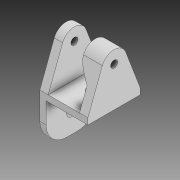
# Autodesk Inventor part: ZIdler
Saved by Autodesk Inventor 2020 (Build 240168000, 168)
## iProperties
Created: 2020-10-21
Part Number: ZIdler
Material: Generic
Document SubType Name: Modeling
Designer: DDeGo
Density: 1 g/cm^3
Appearance: Default
Author: DDeGo
Autodesk Inventor part; units mm, degrees
ref_plane "YZ Plane" through (0, 0, 0) normal (1, 0, 0) x (0, 1, 0)
ref_plane "XZ Plane" through (0, 0, 0) normal (0, 1, 0) x (-1, 0, 0)
ref_plane "XY Plane" through (0, 0, 0) normal (0, 0, 1) x (1, 0, 0)
sketch "Sketch1" plane through (0, 0, 0) normal (0, 0, 1) x (1, 0, 0)
  line L0 (0, 0) -> (23, 0)
  line L1 (23, 0) -> (23, -3)
  line L2 (23, -3) -> (3, -3)
  line L3 (3, -3) -> (3, -23)
  line L4 (3, -23) -> (0, -23)
  line L5 (0, -23) -> (0, 0)
  dimension "d0" = 3
  dimension "d1" = 20
  constraints: 12 end point, 7 perpendicular, 1 horizontal
  measures "d0" distance of L0.end L1.end
  measures "d1" distance of L1.end L2.end
extrude "Extrusion1" add sketch "Sketch1" along normal mid plane 25
sketch "Sketch2" plane through (0, 0, 12.5) normal (0, 1, 0) x (1, 0, 0)
  line L0 (23, 25) -> (23, 0) projected
  line L1 (23, 12.5) -> (13, 12.5) construction
  circle A0 centre (13, 12.5) radius 2.75
  line L2 (3, 25) -> (3, 0) projected
  dimension "d14" = 10
  dimension "d15" = 5.5
  constraints: 2 end point, 1 centre point, 1 coincident, 1 horizontal, 1 midpoint
  measures "d14" distance from line of L2 L1.end
  measures "d15" diameter of A0
extrude "Extrusion2" cut sketch "Sketch2" against normal through all
sketch "Sketch3" plane through (0, -23, 12.5) normal (-1, 0, 0) x (0, 0, 1)
  line L0 (-25, 0) -> (0, 0) projected
  line L1 (-12.5, 0) -> (-12.5, 10) construction
  circle A0 centre (-12.5, 10) radius 2.75
  line L2 (-25, 20) -> (0, 20) projected
  point P0 (-12.5, 23)
  dimension "d10" = 10
  dimension "d11" = 5.5
  constraints: 2 end point, 1 centre point, 1 coincident, 1 midpoint, 1 vertical
  measures "d10" distance from line of L1.end L2
  measures "d11" diameter of A0
extrude "Extrusion3" cut sketch "Sketch3" against normal through all
sketch "Sketch5" plane through (0, -23, 12.5) normal (-1, 0, 0) x (0, 0, 1)
  line L0 (-12.5, 23) -> (-12.5, 39) construction
  arc A0 (-6.8914, 41.1317) -> (-18.1086, 41.1317) centre (-12.5, 39) ccw
  circle A1 centre (-12.5, 39) radius 1.65
  line L1 (-25, 23) -> (0, 23) projected
  line L2 (-25, 23) -> (-18.1086, 41.1317)
  line L3 (-6.8914, 41.1317) -> (0, 23)
  line L4 (0, 23) -> (-25, 23)
  dimension "d23" = 3.3
  dimension "d24" = 12
  dimension "d25" = 16
  constraints: 8 end point, 2 centre point, 2 coincident, 2 point on circle, 2 tangent, 1 collinear, 1 vertical
  measures "d23" diameter of A1
  measures "d24" diameter of A0
  measures "d25" distance of L0.start L0.end
extrude "Extrusion5" add sketch "Sketch5" against normal blind 4
sketch "Sketch6" plane through (23, -3, 12.5) normal (1, 0, 0) x (0, 0, -1)
  line L0 (6.8914, 21.1317) -> (0, 3) projected
  line L1 (25, 3) -> (0, 3) projected
  line L2 (25, 3) -> (18.1086, 21.1317) projected
  arc A0 (18.1086, 21.1317) -> (6.8914, 21.1317) centre (12.5, 19) ccw projected
  circle A1 centre (12.5, 19) radius 1.65 projected
  point P0 (12.5, 3)
extrude "Extrusion6" add sketch "Sketch6" against normal blind 4
fillet "Fillet1" radius 10 2 edges at (1.5, -23, 12.5) (1.5, -23, -12.5)
ref_plane "Work Plane2" through (14, -23, 12.5) normal (1, 0, 0) x (0, 0, -1)
sketch "Sketch7" plane through (19, -3, 12.5) normal (-1, 0, 0) x (0, 0, 1)
  circle A0 centre (-12.5, 19) radius 1.65 projected
  arc A1 (-6.8914, 21.1317) -> (-18.1086, 21.1317) centre (-12.5, 19) ccw projected
  circle A2 centre (-12.5, 19) radius 6
  point P0 (-12.5, 3)
  constraints: 1 coincident, 3 other
extrude "Extrusion7" add sketch "Sketch7" along normal up to surface (5 mm away)
chamfer "Chamfer1" distance 5 angle 45 1 edges at (19, 10, 0)
body "Solid1"
